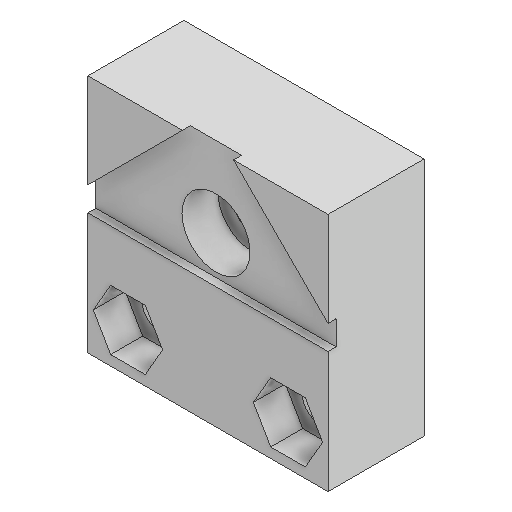
# Autodesk Inventor part: 210505 - Prism adapter v3
Saved by Autodesk Inventor 2022 (Build 260153000, 153)
## iProperties
Created: 2021-05-14
Part Number: 210505 - Prism adapter v3
Material: Generic
Document SubType Name: Modeling
Designer: Ralf
Density: 1 g/cm^3
Appearance: Default
Author: Ralf
Autodesk Inventor part; units mm, degrees
ref_plane "YZ Plane" through (0, 0, 0) normal (1, 0, 0) x (0, 1, 0)
ref_plane "XZ Plane" through (0, 0, 0) normal (0, 1, 0) x (-1, 0, 0)
ref_plane "XY Plane" through (0, 0, 0) normal (0, 0, 1) x (1, 0, 0)
sketch "Sketch1" plane through (0, 0, 0) normal (0, 0, 1) x (1, 0, 0)
  line L0 (-15, 15) -> (15, 15)
  line L1 (15, 15) -> (15, -15)
  line L2 (15, -15) -> (-15, -15)
  line L3 (-15, -15) -> (-15, 15)
  point P0 (0, 0)
  dimension "d0" = 30
  dimension "d1" = 30
  dimension "d2" = 15
  dimension "d3" = 15
  constraints: 8 end point, 2 parallel, 1 horizontal, 1 perpendicular
  measures "d0" distance of L0.start L0.end
  measures "d1" distance of L0.end L1.end
  measures "d2" distance from line of point (0, 0) L2
  measures "d3" distance from line of point (0, 0) L1
extrude "Extrusion1" add sketch "Sketch1" along normal blind 12
sketch "Sketch2" plane through (0, 0, 12) normal (0, 0, 1) x (1, 0, 0)
  circle A0 centre (0, 5) radius 2.25
  line L0 (15, 15) -> (-15, 15) projected
  dimension "d34" = 4.5
  dimension "d35" = 10
  constraints: 1 centre point
  measures "d34" diameter of A0
  measures "d35" distance from line of L0 A0.centre
extrude "Extrusion2" cut sketch "Sketch2" against normal blind 12
sketch "Sketch3" plane through (0, 0, 12) normal (0, 0, 1) x (1, 0, 0)
  circle A0 centre (0, 5) radius 4.25
  line L0 (15, 15) -> (-15, 15) projected
  dimension "d32" = 8.5
  dimension "d33" = 10
  constraints: 1 centre point
  measures "d32" diameter of A0
  measures "d33" distance from line of L0 A0.centre
extrude "Extrusion3" cut sketch "Sketch3" against normal blind 5.5
sketch "Sketch4" plane through (0, 0, 12) normal (0, 0, 1) x (1, 0, 0)
  line L0 (0, 0) -> (0, 18.2)
  line L1 (0, 18.2) -> (-18.0312, 0.1688)
  line L2 (0, 18.2) -> (18.0312, 0.1688)
  line L3 (0, 18.2) -> (25.5, 18.2) construction
  line L4 (18.0312, 0.1688) -> (-18.0312, 0.1688)
  dimension "d12" = 18.2
  dimension "d13" = 25.5
  dimension "d14" = 45
  dimension "d26" = 25.5
  dimension "d27" = 45
  constraints: 10 end point, 1 equal length, 1 horizontal, 1 vertical
  measures "d12" distance of L0.start L0.end
  measures "d13" distance of L0.end L1.end
  measures "d14" angle of L1 L0
  measures "d26" distance of L0.end L2.end
  measures "d27" angle of L2 L3
extrude "Extrusion4" cut sketch "Sketch4" against normal blind 1
sketch "Sketch5" plane through (0, 0, 12) normal (0, 0, 1) x (1, 0, 0)
  circle A0 centre (10, -10) radius 2.25
  line L0 (-15, -15) -> (15, -15) projected
  line L1 (15, -15) -> (15, 15) projected
  circle A1 centre (-10, -10) radius 2.25
  line L2 (-15, 0.1688) -> (-15, -15) projected
  point P0 (0, 0)
  point P1 (15, 0.3223)
  point P2 (-15, 0.3223)
  dimension "d18" = 4.5
  dimension "d19" = 5
  dimension "d20" = 5
  dimension "d21" = 4.5
  dimension "d22" = 5
  dimension "d23" = 5
  constraints: 2 centre point
  measures "d18" diameter of A0
  measures "d19" distance from line of L0 A0.centre
  measures "d20" distance from line of L1 A0.centre
  measures "d21" diameter of A1
  measures "d22" distance from line of L0 A1.centre
  measures "d23" distance from line of A1.centre L2
extrude "Extrusion5" cut sketch "Sketch5" against normal blind 12
sketch "Sketch6" plane through (0, 0, 12) normal (0, 0, 1) x (1, 0, 0)
  circle A0 centre (-10, -10) radius 2.25 projected
  line L0 (-12.1651, -13.75) -> (-14.3301, -10)
  line L1 (-14.3301, -10) -> (-12.1651, -6.25)
  line L2 (-12.1651, -6.25) -> (-7.8349, -6.25)
  line L3 (-7.8349, -6.25) -> (-5.6699, -10)
  line L4 (-5.6699, -10) -> (-7.8349, -13.75)
  line L5 (-7.8349, -13.75) -> (-12.1651, -13.75)
  circle A1 centre (10, -10) radius 2.25 projected
  line L6 (7.8349, -13.75) -> (5.6699, -10)
  line L7 (5.6699, -10) -> (7.8349, -6.25)
  line L8 (7.8349, -6.25) -> (12.1651, -6.25)
  line L9 (12.1651, -6.25) -> (14.3301, -10)
  line L10 (14.3301, -10) -> (12.1651, -13.75)
  line L11 (12.1651, -13.75) -> (7.8349, -13.75)
  point P0 (0, 0)
  dimension "d28" = 7.5
  dimension "d29" = 7.5
  constraints: 24 end point, 2 coincident, 26 other
  measures "d28" distance between parallel lines of L5 L2
  measures "d29" distance between parallel lines of L11 L8
extrude "Extrusion6" cut sketch "Sketch6" against normal blind 4
body "Solid1"
